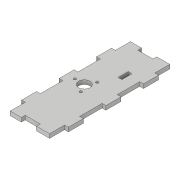
# Autodesk Inventor part: costat3
Saved by Autodesk Inventor 2019 (Build 230136000, 136)
## iProperties
Created: 2018-09-21
Part Number: costat3
Material: Genérico
Document SubType Name: Modeling
Designer: lmacia
Density: 1 g/cm^3
Appearance: Valor por defecto
Author: lmacia
Autodesk Inventor part; units mm, degrees
ref_plane "YZ Plane" through (0, 0, 0) normal (1, 0, 0) x (0, 1, 0)
ref_plane "XZ Plane" through (0, 0, 0) normal (0, 1, 0) x (-1, 0, 0)
ref_plane "XY Plane" through (0, 0, 0) normal (0, 0, 1) x (1, 0, 0)
sketch "Boceto1" plane through (0, 0, 0) normal (0, 1, 0) x (-1, 0, 0)
  line L0 (-13.9366, -26.8506) -> (-11.6866, -26.8506)
  line L1 (-11.6866, -26.8506) -> (-11.6866, -35.7756)
  line L2 (-11.6866, -35.7756) -> (-3.9241, -35.7756)
  line L3 (-3.9241, -35.7756) -> (-3.9241, -33.5256)
  line L4 (-3.9241, -33.5256) -> (5.0759, -33.5256)
  line L5 (5.0759, -33.5256) -> (5.0759, -35.7756)
  line L6 (5.0759, -35.7756) -> (6.7964, -35.7756)
  line L7 (6.7964, -35.7756) -> (11.7134, -35.7756)
  line L8 (11.7134, -35.7756) -> (11.7134, -35.375)
  line L9 (11.7134, -35.375) -> (11.7134, -33.5256)
  line L10 (11.7134, -33.5256) -> (11.7134, -26.8257)
  line L11 (11.7134, -26.8257) -> (13.9634, -26.8257)
  line L12 (13.9634, -26.8257) -> (13.9634, -17.8506)
  line L13 (13.9637, -17.8506) -> (11.7151, -17.8506)
  line L14 (11.7151, -17.8506) -> (11.7144, -7.4795)
  line L15 (11.7144, -7.4795) -> (11.7134, -4.5006)
  line L16 (11.7118, -4.5504) -> (11.7134, -4.5006)
  line L17 (11.7134, -4.5006) -> (13.9634, -4.5006)
  line L18 (13.9634, -4.5006) -> (13.9634, 4.4994)
  line L19 (13.9634, 4.4994) -> (11.7134, 4.4994)
  line L20 (11.7134, 4.4994) -> (11.7134, 17.8494)
  line L21 (11.7134, 17.8494) -> (13.9634, 17.8494)
  line L22 (13.9634, 17.8494) -> (13.9634, 26.8494)
  line L23 (13.9634, 26.8494) -> (11.7134, 26.8494)
  line L24 (11.7134, 26.8494) -> (11.7134, 33.5244)
  line L25 (11.7134, 33.5244) -> (11.7134, 35.7744)
  line L26 (11.7134, 35.7744) -> (5.0759, 35.7744)
  line L27 (5.0759, 35.7744) -> (5.0759, 33.5244)
  line L28 (5.0759, 33.5244) -> (-2.6866, 33.5244)
  line L29 (-2.6866, 33.5244) -> (-3.9241, 33.5244)
  line L30 (-3.9241, 33.5244) -> (-3.9241, 35.7744)
  line L31 (-3.9241, 35.7744) -> (-11.6866, 35.7744)
  line L32 (-11.6866, 35.7744) -> (-11.6866, 26.8494)
  line L33 (-11.6866, 26.8494) -> (-13.9366, 26.8494)
  line L34 (-13.9366, 26.8494) -> (-13.9366, 17.8494)
  line L35 (-13.9366, 17.8494) -> (-11.6866, 17.8494)
  line L36 (-11.6866, 17.8494) -> (-11.6866, 4.4994)
  line L37 (-11.6866, 4.4994) -> (-13.9366, 4.4994)
  line L38 (-13.9366, 4.4994) -> (-13.9366, -4.5006)
  line L39 (-13.9366, -4.5006) -> (-11.6866, -4.5006)
  line L40 (-11.6866, -4.5006) -> (-11.6866, -17.8506)
  line L41 (-11.6866, -17.8506) -> (-13.1866, -17.8506)
  line L42 (-13.1866, -17.8506) -> (-13.9366, -17.8506)
  line L43 (-13.9366, -17.8506) -> (-13.9366, -26.8506)
  line L44 (-12.075, -17.85) -> (-14.325, -17.85)
  line L45 (4.6875, 33.525) -> (3.4125, 33.525)
  line L46 (-3.075, -13.65) -> (-3.075, -19.65)
  line L47 (-3.075, -19.65) -> (-5.325, -19.65)
  line L48 (-5.325, -19.65) -> (-5.325, -13.65)
  line L49 (-5.325, -13.65) -> (-3.075, -13.65)
  circle A0 centre (0.6, 4.875) radius 0.75
  circle A1 centre (3.375, 0) radius 3.375
  circle A2 centre (9, 0) radius 0.75
  circle A3 centre (0.6, -4.875) radius 0.75
  point P0 (0, 0)
  constraints: 100 end point, 4 centre point, 1 horizontal, 1 point on line
extrude "Extrusión1" add sketch "Boceto1" along normal blind 2.4
